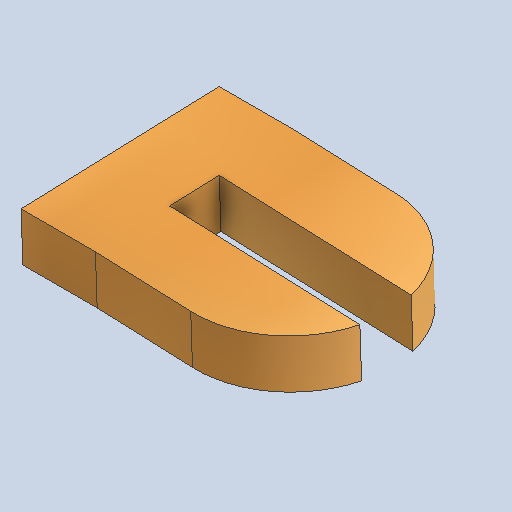
# Autodesk Inventor part: aux_nose_side_bracket
Saved by Autodesk Inventor 2022 (Build 260153070, 153G)
## iProperties
Created: 2021-04-29
Part Number: aux_nose_side_bracket
Material: Plywood, Sheathing, Glazed
Document SubType Name: Modeling
Designer: kardo
Density: 0.75 g/cm^3
Appearance: Plywood - New(2)
Mass: 0.0991298 g
Surface Area: 2.33959 cm^2
Volume: 0.132173 cm^3
Author: kardo
Autodesk Inventor part; units mm, degrees
ref_plane "YZ Plane" through (0, 0, 0) normal (1, 0, 0) x (0, 1, 0)
ref_plane "XZ Plane" through (0, 0, 0) normal (0, 1, 0) x (-1, 0, 0)
ref_plane "XY Plane" through (0, 0, 0) normal (0, 0, 1) x (1, 0, 0)
derived "frame_outline.ipt"
sketch "joints" plane through (81, 0, 0) normal (1, 0, 0) x (0, 1, 0)
  line L0 (-37.9005, 25.6108) -> (-277.6703, 19.7906) construction
  line L1 (94.8, 28.832) -> (28.4595, 27.2216) construction
  line L2 (28.4595, 27.2216) -> (-37.9005, 25.6108) construction
  line L3 (-363, 18.496) -> (-297.6664, 19.4083) construction
  line L4 (-121, 716.7765) -> (-121, -158.9765) construction
  line L5 (-242, 716.7765) -> (-242, -158.9765) construction
  line L6 (237, 716.7765) -> (237, -158.9765) construction
  line L7 (-363, 716.7765) -> (-363, -158.9765) construction
  line L8 (143.2909, -175.9483) -> (77.9563, 758.3799) construction
  line L9 (0, 0) -> (130.35, 9.115) construction
  line L10 (0, 716.7765) -> (0, -158.9765) construction
  line L11 (-242, 46.7048) -> (-242, 33.6806) construction
  line L12 (-242, 33.6806) -> (-242, 20.6564) construction
  line L13 (-363, 38.08) -> (-363, 28.288) construction
  line L14 (-363, 28.288) -> (-363, 18.496) construction
  line L15 (-121, 51.5188) -> (-121, 37.5562) construction
  line L16 (-121, 37.5562) -> (-121, 23.5936) construction
  line L17 (0, 54.4) -> (0, 40.4654) construction
  line L18 (0, 40.4654) -> (0, 26.5308) construction
  line L19 (94.8, 37.536) -> (94.8, 33.184) construction
  line L20 (94.8, 33.184) -> (94.8, 28.832) construction
  line L21 (94.8, 37.536) -> (94.8, 28.832) construction
  line L22 (130.35, 9.115) -> (129.7793, 17.2757) construction
  line L23 (129.7793, 17.2757) -> (129.2087, 25.4364) construction
  line L24 (129.2087, 25.4364) -> (128.638, 33.5972) construction
  line L25 (128.638, 33.5972) -> (128.0674, 41.7579) construction
  line L26 (128.0674, 41.7579) -> (127.4967, 49.9186) construction
  spline S0 degree 3 poles (-363, 38.08) (-277.2033, 46.9603) (-131.9759, 52.0964) (0, 54.4) knots 0 0 0 0 1 1 1 1 construction
  spline S1 degree 3 poles (-297.6664, 19.4083) (-291.0004, 19.5014) (-284.3349, 19.6288) (-277.6703, 19.7906) knots 0 0 0 0 1 1 1 1 construction
  spline S2 degree 4 poles (0, 54.4) (23.3745, 54.808) (84.9613, 55.883) (149.0088, 47.5461) (201.9993, 42.6196) (237, 36.448) knots 0 0 0 0 0 0.379537 1 1 1 1 1 construction
  spline S3 degree 3 poles (130.35, 9.115) (172.0992, 12.0344) (220.2053, 21.9532) (237, 36.448) knots 0 0 0 0 1 1 1 1 construction
sketch "joints_nose" plane through (84, 0, 0) normal (1, 0, 0) x (0, 1, 0)
  line L0 (129.046, 27.7634) -> (235.7442, 35.2245) construction
  line L1 (128.6952, 32.7794) -> (236.1697, 36.5325) construction
  line L2 (195.9322, 35.1273) -> (196.0258, 32.4471) construction
  line L3 (196.2351, 29.4544) -> (196.0258, 32.4471)
  line L4 (196.0258, 32.4471) -> (195.8863, 34.4422)
  line L5 (195.8863, 34.4422) -> (195.677, 37.4349)
  line L6 (203.8226, 38.4047) -> (203.9273, 35.4065)
  line L7 (203.9971, 33.4077) -> (204.1018, 30.4096)
  line L8 (203.9273, 35.4065) -> (203.9971, 33.4077)
  point P0 (0, 0)
ref_plane "plane_sponson_edge_side" through (81, 0, 28.1718) normal (0.0377663, 0.0348746, -0.9986779) x (0, 0.9993908, 0.0348995)
ref_plane "plane_stringer_outer" through (84, 0, 0) normal (1, 0, 0) x (0, 1, 0)
sketch "Sketch3" plane through (84, 0, 0) normal (1, 0, 0) x (0, 1, 0)
  line L0 (204.1018, 30.4096) -> (203.8226, 38.4047)
  line L1 (203.8226, 38.4047) -> (201.8239, 38.3349)
  line L2 (201.8239, 38.3349) -> (202.103, 30.3398)
  line L3 (202.103, 30.3398) -> (204.1018, 30.4096)
  point P0 (0, 0)
  dimension "d10" = 2
  constraints: 8 end point, 2 parallel, 1 perpendicular
  measures "d10" distance of L0.end L1.end
extrude "Extrusion1" add sketch "Sketch3" against normal blind 3
sketch "Sketch6" plane through (81, 204.1018, 30.4096) normal (0, 0.9993908, 0.0348995) x (1, 0, 0)
  line L0 (3, 0) -> (3, -8) projected
  line L1 (3, 0) -> (0, 0) projected
  line L2 (0, -8) -> (0, 0) projected
  line L3 (3, -8) -> (0, -8) projected
  line L4 (-101.3104, -1.0578) -> (32.0227, -6.0969) projected
  line L5 (3, 0) -> (3, -8) projected
  line L6 (3, -8) -> (10.9943, -8.3021)
  line L7 (10.9943, -8.3021) -> (11.2962, -0.3135)
  line L8 (11.2962, -0.3135) -> (3, 0)
  point P0 (-81, 23.268)
  constraints: 6 end point, 2 parallel, 1 equal length, 1 perpendicular
extrude "Extrusion4" add sketch "Sketch6" against normal up to surface (2 mm away) contours L8 L7 L4 L0 | L4 L7 L6 L0
full round fillet "Full Round Fillet2" first side at (89.3295, 202.4831, 38.5595) centre faces at (92.0949, 202.5725, 35.9989) second side at (89.5308, 203.4283, 30.5952)
sketch "Sketch7" plane through (81, 204.1018, 30.4096) normal (0, 0.9993908, 0.0348995) x (1, 0, 0)
  line L0 (-101.3104, -1.0578) -> (32.0227, -6.0969) projected
  arc A0 (7, -8.1512) -> (7.3019, -0.1626) centre (7.151, -4.1569) ccw projected
  line L1 (11.0558, -3.303) -> (3, -2.9986)
  line L2 (3, -2.9986) -> (3, -5)
  point P0 (-81, 23.268)
  point P1 (3, -8)
  point P2 (3, 0)
  point P3 (10.9807, -5.3016)
  dimension "d14" = 2
  constraints: 4 end point, 3 point on line, 1 parallel, 1 point on circle
  measures "d14" distance between parallel lines of L0 L1
extrude "Extrusion5" cut sketch "Sketch7" along normal through all both and the other way through all
equation "\"d10\" = bulkhead_thickness"
equation "\"d3\" = stringer_thickness"
equation "\"d11\" = stringer_thickness"
equation "\"d14\" = bulkhead_thickness"
equation "\"bulkhead_thickness\" = 2"
equation "\"stringer_thickness\" = 3"
body "Solid1"
